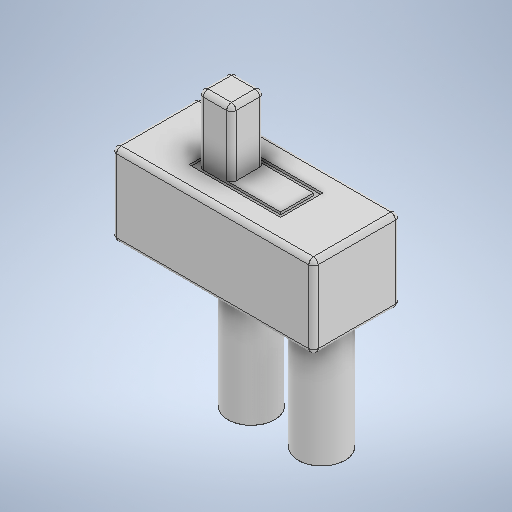
# Autodesk Inventor part: Schalter
Saved by Autodesk Inventor 2025.2 (Build 292293000, 293)
## iProperties
Created: 2024-11-18
Part Number: Schalter
Material: Generisch
Document SubType Name: Modeling
Designer: tills
Density: 1 g/cm^3
Appearance: Vorgabe
Author: tills
Autodesk Inventor part; units mm, degrees
ref_plane "YZ Plane" through (0, 0, 0) normal (1, 0, 0) x (0, 1, 0)
ref_plane "XZ Plane" through (0, 0, 0) normal (0, 1, 0) x (-1, 0, 0)
ref_plane "XY Plane" through (0, 0, 0) normal (0, 0, 1) x (1, 0, 0)
sketch "Skizze1" plane through (0, 0, 0) normal (0, 1, 0) x (-1, 0, 0)
  line L0 (4.3, 1.85) -> (-4.3, 1.85)
  line L1 (-4.3, 1.85) -> (-4.3, -1.85)
  line L2 (-4.3, -1.85) -> (4.3, -1.85)
  line L3 (4.3, -1.85) -> (4.3, 1.85)
  line L4 (4.3, 1.85) -> (-4.3, -1.85) construction
  line L5 (-4.3, 1.85) -> (4.3, -1.85) construction
  point P0 (0, 0)
  dimension "d0" = 8.6
  dimension "d1" = 3.7
  constraints: 12 end point, 2 midpoint, 2 parallel, 1 horizontal, 1 perpendicular
  measures "d0" distance of L1.end L2.end
  measures "d1" distance of L0.end L1.end
extrude "Extrusion1" add sketch "Skizze1" along normal blind 3.5
sketch "Skizze2" plane through (0, 3.5, 0) normal (0, 1, 0) x (1, 0, 0)
  line L0 (-1.75, -0.7) -> (1.75, -0.7)
  line L1 (1.75, -0.7) -> (1.75, 0.7)
  line L2 (1.75, 0.7) -> (-1.75, 0.7)
  line L3 (-1.75, 0.7) -> (-1.75, -0.7)
  line L4 (-1.75, -0.7) -> (1.75, 0.7) construction
  line L5 (1.75, -0.7) -> (-1.75, 0.7) construction
  line L6 (-1.95, -0.9) -> (1.95, -0.9)
  line L7 (1.95, -0.9) -> (1.95, 0.9)
  line L8 (1.95, 0.9) -> (-1.95, 0.9)
  line L9 (-1.95, 0.9) -> (-1.95, -0.9)
  line L10 (-1.95, -0.9) -> (1.95, 0.9) construction
  line L11 (1.95, -0.9) -> (-1.95, 0.9) construction
  point P0 (0, 0)
  dimension "d4" = 1.4
  dimension "d5" = 3.5
  dimension "d6" = 0.2
  dimension "d7" = 0.2
  constraints: 24 end point, 4 midpoint, 4 parallel, 2 horizontal, 2 perpendicular
  measures "d4" distance of L0.end L1.end
  measures "d5" distance of L1.end L2.end
  measures "d6" distance between parallel lines of L7 L1
  measures "d7" distance between parallel lines of L2 L8
extrude "Extrusion2" cut sketch "Skizze2" against normal blind 0.1
sketch "Skizze3" plane through (0, 3.5, 0) normal (0, 1, 0) x (1, 0, 0)
  line L0 (-1.75, 0.7) -> (-1.75, -0.7) projected
  line L1 (1.75, 0.7) -> (-1.75, 0.7) projected
  line L2 (-1.75, -0.7) -> (1.75, -0.7) projected
  line L3 (-1.75, 0.7) -> (-0.35, 0.7)
  line L4 (-0.35, 0.7) -> (-0.35, -0.7)
  line L5 (-0.35, -0.7) -> (-1.75, -0.7)
  line L6 (-1.75, -0.7) -> (-1.75, 0.7)
  point P0 (0, 0)
  dimension "d10" = 1.4
  constraints: 8 end point, 2 parallel, 1 horizontal, 1 perpendicular, 1 point on line
  measures "d10" distance between parallel lines of L0 L4
extrude "Extrusion3" add sketch "Skizze3" along normal blind 2.8
sketch "Skizze4" plane through (0, 0, 0) normal (0, -1, 0) x (1, 0, 0)
  circle A0 centre (-0.2, 0) radius 1
  circle A1 centre (2.8, 0) radius 1
  line L0 (4.3, 1.85) -> (4.3, -1.85) projected
  point P0 (0, 0)
  dimension "d16" = 1.5
  dimension "d17" = 3
  dimension "d18" = 2
  constraints: 2 centre point, 1 equal radius
  measures "d16" distance from line of L0 A1.centre
  measures "d17" distance of A0.centre A1.centre
  measures "d18" diameter of A1
extrude "Extrusion4" add sketch "Skizze4" along normal blind 5
fillet "Rundung1" radius 0.2 20 edges at (0, 3.5, 1.85) (4.3, 3.5, 0) (4.3, 1.75, 1.85) (4.3, 0, 0) (4.3, 1.75, -1.85) (0, 3.5, -1.85) (0, 0, -1.85) (-4.3, 1.75, -1.85) (-4.3, 0, 0) (-4.3, 1.75, 1.85) (-4.3, 3.5, 0) (0, 0, 1.85) (-0.35, 4.9, -0.7) (-1.75, 4.85, -0.7) (-1.75, 4.85, 0.7) (-0.35, 4.9, 0.7) (-1.05, 6.3, 0.7) (-0.35, 6.3, 0) (-1.05, 6.3, -0.7) (-1.75, 6.3, 0)
chamfer "Fasen1" distance 0.2 angle 45 2 edges at (-1.2, 0, 0) (1.8, 0, 0)
